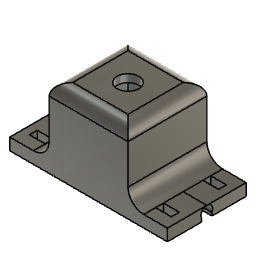
led case v2 (Autodesk Fusion 360 design; units mm, degrees)
Autodesk Fusion 360 part; units mm, degrees
box "PrimitivaParallelepipedo1" add length 20 width 20 height 20 placed x (0, 1, 0) y (-1, 0, 0) z (0, 0, 1) at (20, 0, 0)
shell "Svuotamento1" thickness 2 removed faces 1 at (6.6667, 6.6667, 0)
box "PrimitivaParallelepipedo2" add length 20 width 10 height 3 placed x (0, 1, 0) y (-1, 0, 0) z (0, 0, 1) at (30, 0, 0)
box "PrimitivaParallelepipedo3" add length 20 width 10 height 3 placed x (0, 1, 0) y (-1, 0, 0) z (0, 0, 1) at (0, 0, 0)
cylinder "PrimitivaCilindro1" cut diameter 5.5 height 50 placed x (1, 0, 0) y (0, 1, 0) z (0, 0, 1) at (10, 10, 0)
fillet "Raccordo1" radius 4 1 edges at (20, 10, 3)
fillet "Raccordo2" radius 4 1 edges at (0, 10, 3)
fillet "Raccordo3" radius 3 4 edges at (20, 10, 20) (10, 20, 20) (0, 10, 20) (10, 0, 20)
fillet "Raccordo4" radius 3 4 edges at (10, 2, 18) (2, 10, 18) (10, 18, 18) (18, 10, 18)
sketch "Schizzo5" plane through (2, 0, 0) normal (1, 0, 0) x (0, 1, 0)
  line L0 (18, 15) -> (2, 15)
  line L1 (2, 15) -> (2, 0)
  line L2 (2, 0) -> (18, 0)
  line L3 (18, 0) -> (18, 15)
box "PrimitivaParallelepipedo4" cut length 2 width 4 height -41 placed x (0, 1, 0) y (-1, 0, 0) z (0, 0, 1) at (28, 15, 20)
box "PrimitivaParallelepipedo5" cut length 2 width 4 height 6 placed x (0, 1, 0) y (-1, 0, 0) z (0, 0, 1) at (28, 3, 0)
box "PrimitivaParallelepipedo6" cut length 2 width 4 height 8 placed x (0, -1, 0) y (1, 0, 0) z (0, 0, 1) at (-8, 17, 0)
box "PrimitivaParallelepipedo7" cut length 2 width 4 height -45 placed x (0, -1, 0) y (1, 0, 0) z (0, 0, 1) at (-8, 5, 20)
cylinder "PrimitivaCilindro2" cut diameter 3 height -44 placed x (0, 0, 1) y (0, 1, 0) z (-1, 0, 0) at (-10, 10, 1.5)
box "PrimitivaParallelepipedo8" cut length 0.872 width 2.6784 height -43 placed x (0, 0, 1) y (0, 1, 0) z (-1, 0, 0) at (-10, 8.6378, 0)
